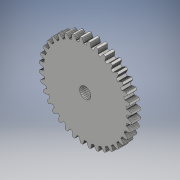
# Autodesk Inventor part: Engranajes GRANDE final 2017
Saved by Autodesk Inventor 2017 (Build 210142000, 142)
## iProperties
Created: 2017-09-25
Part Number: Engranajes GRANDE final 2017
Material: Generic
Document SubType Name: Modeling
Designer: ANDRES
Density: 1 g/cm^3
Appearance: Default
Author: ANDRES
Autodesk Inventor part; units mm, degrees
(part 1 of 2)
ref_plane "YZ Plane" through (0, 0, 0) normal (1, 0, 0) x (0, 1, 0)
ref_plane "XZ Plane" through (0, 0, 0) normal (0, 1, 0) x (-1, 0, 0)
ref_plane "XY Plane" through (0, 0, 0) normal (0, 0, 1) x (1, 0, 0)
sketch "Sketch1" plane through (0, 0, 0) normal (0, 1, 0) x (-1, 0, 0)
  line L0 (23.3143, 11.8442) -> (23.3436, 11.8386)
  line L1 (23.3436, 11.8386) -> (23.3729, 11.8325)
  line L2 (23.3729, 11.8325) -> (23.4022, 11.8259)
  line L3 (23.4022, 11.8259) -> (23.4314, 11.8189)
  line L4 (23.4314, 11.8189) -> (23.4899, 11.8037)
  line L5 (23.4899, 11.8037) -> (23.5482, 11.7869)
  line L6 (23.5482, 11.7869) -> (23.6648, 11.7495)
  line L7 (23.6648, 11.7495) -> (23.781, 11.7072)
  line L8 (23.781, 11.7072) -> (23.8968, 11.6604)
  line L9 (23.8968, 11.6604) -> (24.0123, 11.6095)
  line L10 (24.0123, 11.6095) -> (24.1274, 11.5547)
  line L11 (24.1274, 11.5547) -> (24.2421, 11.4962)
  line L12 (24.2421, 11.4962) -> (24.3563, 11.434)
  line L13 (24.3563, 11.434) -> (24.47, 11.3684)
  line L14 (24.47, 11.3684) -> (24.4188, 10.8271)
  line L15 (24.4188, 10.8271) -> (24.2948, 10.784)
  line L16 (24.2948, 10.784) -> (24.171, 10.7443)
  line L17 (24.171, 10.7443) -> (24.0474, 10.7083)
  line L18 (24.0474, 10.7083) -> (23.9241, 10.676)
  line L19 (23.9241, 10.676) -> (23.8011, 10.6477)
  line L20 (23.8011, 10.6477) -> (23.6785, 10.6234)
  line L21 (23.6785, 10.6234) -> (23.5564, 10.6037)
  line L22 (23.5564, 10.6037) -> (23.435, 10.5887)
  line L23 (23.435, 10.5887) -> (23.3745, 10.5832)
  line L24 (23.3745, 10.5832) -> (23.3142, 10.5792)
  line L25 (23.3142, 10.5792) -> (23.2842, 10.5778)
  line L26 (23.2842, 10.5778) -> (23.2542, 10.5768)
  line L27 (23.2542, 10.5768) -> (23.2243, 10.5763)
  line L28 (23.2243, 10.5763) -> (23.1944, 10.5763)
  line L29 (23.1944, 10.5763) -> (23.0757, 9.9292)
  line L30 (23.0757, 9.9292) -> (23.1036, 9.9186)
  line L31 (23.1036, 9.9186) -> (23.1314, 9.9075)
  line L32 (23.1314, 9.9075) -> (23.159, 9.896)
  line L33 (23.159, 9.896) -> (23.1866, 9.884)
  line L34 (23.1866, 9.884) -> (23.2415, 9.8588)
  line L35 (23.2415, 9.8588) -> (23.2961, 9.8322)
  line L36 (23.2961, 9.8322) -> (23.4044, 9.7751)
  line L37 (23.4044, 9.7751) -> (23.5115, 9.7133)
  line L38 (23.5115, 9.7133) -> (23.6174, 9.6472)
  line L39 (23.6174, 9.6472) -> (23.7223, 9.577)
  line L40 (23.7223, 9.577) -> (23.8262, 9.503)
  line L41 (23.8262, 9.503) -> (23.9289, 9.4254)
  line L42 (23.9289, 9.4254) -> (24.0306, 9.3443)
  line L43 (24.0306, 9.3443) -> (24.1312, 9.26)
  line L44 (24.1312, 9.26) -> (23.9868, 8.7358)
  line L45 (23.9868, 8.7358) -> (23.8572, 8.7148)
  line L46 (23.8572, 8.7148) -> (23.7284, 8.6973)
  line L47 (23.7284, 8.6973) -> (23.6004, 8.6833)
  line L48 (23.6004, 8.6833) -> (23.4733, 8.6729)
  line L49 (23.4733, 8.6729) -> (23.3473, 8.6663)
  line L50 (23.3473, 8.6663) -> (23.2224, 8.6638)
  line L51 (23.2224, 8.6638) -> (23.0987, 8.6655)
  line L52 (23.0987, 8.6655) -> (22.9765, 8.6718)
  line L53 (22.9765, 8.6718) -> (22.916, 8.6769)
  line L54 (22.916, 8.6769) -> (22.856, 8.6834)
  line L55 (22.856, 8.6834) -> (22.8261, 8.6873)
  line L56 (22.8261, 8.6873) -> (22.7964, 8.6915)
  line L57 (22.7964, 8.6915) -> (22.7669, 8.6962)
  line L58 (22.7669, 8.6962) -> (22.7375, 8.7014)
  line L59 (22.7375, 8.7014) -> (22.5082, 8.0848)
  line L60 (22.5082, 8.0848) -> (22.5338, 8.0695)
  line L61 (22.5338, 8.0695) -> (22.5592, 8.0537)
  line L62 (22.5592, 8.0537) -> (22.5845, 8.0375)
  line L63 (22.5845, 8.0375) -> (22.6096, 8.0209)
  line L64 (22.6096, 8.0209) -> (22.6593, 7.9866)
  line L65 (22.6593, 7.9866) -> (22.7084, 7.951)
  line L66 (22.7084, 7.951) -> (22.8051, 7.8759)
  line L67 (22.8051, 7.8759) -> (22.8998, 7.7964)
  line L68 (22.8998, 7.7964) -> (22.9927, 7.7129)
  line L69 (22.9927, 7.7129) -> (23.0838, 7.6255)
  line L70 (23.0838, 7.6255) -> (23.1732, 7.5347)
  line L71 (23.1732, 7.5347) -> (23.2609, 7.4404)
  line L72 (23.2609, 7.4404) -> (23.347, 7.343)
  line L73 (23.347, 7.343) -> (23.4314, 7.2424)
  line L74 (23.4314, 7.2424) -> (23.1982, 6.7513)
  line L75 (23.1982, 6.7513) -> (23.0669, 6.7531)
  line L76 (23.0669, 6.7531) -> (22.937, 6.7582)
  line L77 (22.937, 6.7582) -> (22.8085, 6.7666)
  line L78 (22.8085, 6.7666) -> (22.6816, 6.7786)
  line L79 (22.6816, 6.7786) -> (22.5564, 6.7939)
  line L80 (22.5564, 6.7939) -> (22.4329, 6.8131)
  line L81 (22.4329, 6.8131) -> (22.3114, 6.8362)
  line L82 (22.3114, 6.8362) -> (22.1922, 6.8637)
  line L83 (22.1922, 6.8637) -> (22.1335, 6.8792)
  line L84 (22.1335, 6.8792) -> (22.0755, 6.8961)
  line L85 (22.0755, 6.8961) -> (22.0467, 6.905)
  line L86 (22.0467, 6.905) -> (22.0182, 6.9144)
  line L87 (22.0182, 6.9144) -> (21.9899, 6.9241)
  line L88 (21.9899, 6.9241) -> (21.9619, 6.9343)
  line L89 (21.9619, 6.9343) -> (21.6289, 6.3669)
  line L90 (21.6289, 6.3669) -> (21.6515, 6.3474)
  line L91 (21.6515, 6.3474) -> (21.6738, 6.3275)
  line L92 (21.6738, 6.3275) -> (21.6958, 6.3071)
  line L93 (21.6958, 6.3071) -> (21.7177, 6.2864)
  line L94 (21.7177, 6.2864) -> (21.7607, 6.244)
  line L95 (21.7607, 6.244) -> (21.8029, 6.2003)
  line L96 (21.8029, 6.2003) -> (21.885, 6.1096)
  line L97 (21.885, 6.1096) -> (21.9645, 6.0149)
  line L98 (21.9645, 6.0149) -> (22.0415, 5.9165)
  line L99 (22.0415, 5.9165) -> (22.116, 5.8147)
  line L100 (22.116, 5.8147) -> (22.1883, 5.7097)
  line L101 (22.1883, 5.7097) -> (22.2583, 5.6016)
  line L102 (22.2583, 5.6016) -> (22.3262, 5.4907)
  line L103 (22.3262, 5.4907) -> (22.3918, 5.377)
  line L104 (22.3918, 5.377) -> (22.0769, 4.9338)
  line L105 (22.0769, 4.9338) -> (21.9479, 4.9585)
  line L106 (21.9479, 4.9585) -> (21.8209, 4.986)
  line L107 (21.8209, 4.986) -> (21.6958, 5.0166)
  line L108 (21.6958, 5.0166) -> (21.5729, 5.0503)
  line L109 (21.5729, 5.0503) -> (21.4522, 5.0873)
  line L110 (21.4522, 5.0873) -> (21.3339, 5.1277)
  line L111 (21.3339, 5.1277) -> (21.2183, 5.1716)
  line L112 (21.2183, 5.1716) -> (21.1056, 5.2194)
  line L113 (21.1056, 5.2194) -> (21.0505, 5.2449)
  line L114 (21.0505, 5.2449) -> (20.9963, 5.2715)
  line L115 (20.9963, 5.2715) -> (20.9696, 5.2853)
  line L116 (20.9696, 5.2853) -> (20.9431, 5.2995)
  line L117 (20.9431, 5.2995) -> (20.917, 5.314)
  line L118 (20.917, 5.314) -> (20.8911, 5.3289)
  line L119 (20.8911, 5.3289) -> (20.4647, 4.828)
  line L120 (20.4647, 4.828) -> (20.4835, 4.8049)
  line L121 (20.4835, 4.8049) -> (20.502, 4.7814)
  line L122 (20.502, 4.7814) -> (20.5202, 4.7575)
  line L123 (20.5202, 4.7575) -> (20.5381, 4.7333)
  line L124 (20.5381, 4.7333) -> (20.5731, 4.6841)
  line L125 (20.5731, 4.6841) -> (20.6071, 4.6338)
  line L126 (20.6071, 4.6338) -> (20.6722, 4.5302)
  line L127 (20.6722, 4.5302) -> (20.7341, 4.423)
  line L128 (20.7341, 4.423) -> (20.7928, 4.3127)
  line L129 (20.7928, 4.3127) -> (20.8485, 4.1995)
  line L130 (20.8485, 4.1995) -> (20.9015, 4.0835)
  line L131 (20.9015, 4.0835) -> (20.9517, 3.9649)
  line L132 (20.9517, 3.9649) -> (20.9992, 3.8439)
  line L133 (20.9992, 3.8439) -> (21.0441, 3.7205)
  line L134 (21.0441, 3.7205) -> (20.657, 3.3388)
  line L135 (20.657, 3.3388) -> (20.5343, 3.3854)
  line L136 (20.5343, 3.3854) -> (20.4139, 3.4347)
  line L137 (20.4139, 3.4347) -> (20.2961, 3.4865)
  line L138 (20.2961, 3.4865) -> (20.1809, 3.5411)
  line L139 (20.1809, 3.5411) -> (20.0684, 3.5985)
  line L140 (20.0684, 3.5985) -> (19.959, 3.6587)
  line L141 (19.959, 3.6587) -> (19.8528, 3.722)
  line L142 (19.8528, 3.722) -> (19.7501, 3.7887)
  line L143 (19.7501, 3.7887) -> (19.7002, 3.8233)
  line L144 (19.7002, 3.8233) -> (19.6515, 3.859)
  line L145 (19.6515, 3.859) -> (19.6276, 3.8772)
  line L146 (19.6276, 3.8772) -> (19.604, 3.8957)
  line L147 (19.604, 3.8957) -> (19.5807, 3.9146)
  line L148 (19.5807, 3.9146) -> (19.5578, 3.9338)
  line L149 (19.5578, 3.9338) -> (19.051, 3.5144)
  line L150 (19.051, 3.5144) -> (19.0655, 3.4884)
  line L151 (19.0655, 3.4884) -> (19.0796, 3.462)
  line L152 (19.0796, 3.462) -> (19.0933, 3.4354)
  line L153 (19.0933, 3.4354) -> (19.1068, 3.4084)
  line L154 (19.1068, 3.4084) -> (19.1326, 3.3539)
  line L155 (19.1326, 3.3539) -> (19.1574, 3.2984)
  line L156 (19.1574, 3.2984) -> (19.2036, 3.1851)
  line L157 (19.2036, 3.1851) -> (19.2458, 3.0689)
  line L158 (19.2458, 3.0689) -> (19.2845, 2.9501)
  line L159 (19.2845, 2.9501) -> (19.3198, 2.8289)
  line L160 (19.3198, 2.8289) -> (19.3517, 2.7055)
  line L161 (19.3517, 2.7055) -> (19.3806, 2.58)
  line L162 (19.3806, 2.58) -> (19.4064, 2.4526)
  line L163 (19.4064, 2.4526) -> (19.4292, 2.3233)
  line L164 (19.4292, 2.3233) -> (18.9817, 2.0146)
  line L165 (18.9817, 2.0146) -> (18.8689, 2.0818)
  line L166 (18.8689, 2.0818) -> (18.759, 2.1512)
  line L167 (18.759, 2.1512) -> (18.6519, 2.2227)
  line L168 (18.6519, 2.2227) -> (18.5479, 2.2964)
  line L169 (18.5479, 2.2964) -> (18.4471, 2.3724)
  line L170 (18.4471, 2.3724) -> (18.3498, 2.4507)
  line L171 (18.3498, 2.4507) -> (18.2562, 2.5315)
  line L172 (18.2562, 2.5315) -> (18.1667, 2.615)
  line L173 (18.1667, 2.615) -> (18.1236, 2.6578)
  line L174 (18.1236, 2.6578) -> (18.0818, 2.7013)
  line L175 (18.0818, 2.7013) -> (18.0614, 2.7234)
  line L176 (18.0614, 2.7234) -> (18.0413, 2.7458)
  line L177 (18.0413, 2.7458) -> (18.0217, 2.7684)
  line L178 (18.0217, 2.7684) -> (18.0025, 2.7912)
  line L179 (18.0025, 2.7912) -> (17.4305, 2.4663)
  line L180 (17.4305, 2.4663) -> (17.4403, 2.4381)
  line L181 (17.4403, 2.4381) -> (17.4497, 2.4097)
  line L182 (17.4497, 2.4097) -> (17.4586, 2.381)
  line L183 (17.4586, 2.381) -> (17.4672, 2.3522)
  line L184 (17.4672, 2.3522) -> (17.4832, 2.294)
  line L185 (17.4832, 2.294) -> (17.4979, 2.235)
  line L186 (17.4979, 2.235) -> (17.5237, 2.1154)
  line L187 (17.5237, 2.1154) -> (17.5452, 1.9936)
  line L188 (17.5452, 1.9936) -> (17.5626, 1.8699)
  line L189 (17.5626, 1.8699) -> (17.5763, 1.7445)
  line L190 (17.5763, 1.7445) -> (17.5864, 1.6174)
  line L191 (17.5864, 1.6174) -> (17.593, 1.4888)
  line L192 (17.593, 1.4888) -> (17.5963, 1.3588)
  line L193 (17.5963, 1.3588) -> (17.5963, 1.2275)
  line L194 (17.5963, 1.2275) -> (17.102, 1.0013)
  line L195 (17.102, 1.0013) -> (17.0026, 1.0871)
  line L196 (17.0026, 1.0871) -> (16.9063, 1.1745)
  line L197 (16.9063, 1.1745) -> (16.8133, 1.2636)
  line L198 (16.8133, 1.2636) -> (16.7237, 1.3542)
  line L199 (16.7237, 1.3542) -> (16.6378, 1.4465)
  line L200 (16.6378, 1.4465) -> (16.5555, 1.5406)
  line L201 (16.5555, 1.5406) -> (16.4774, 1.6364)
  line L202 (16.4774, 1.6364) -> (16.4037, 1.7341)
  line L203 (16.4037, 1.7341) -> (16.3687, 1.7838)
  line L204 (16.3687, 1.7838) -> (16.3351, 1.8339)
  line L205 (16.3351, 1.8339) -> (16.3188, 1.8593)
  line L206 (16.3188, 1.8593) -> (16.303, 1.8847)
  line L207 (16.303, 1.8847) -> (16.2876, 1.9104)
  line L208 (16.2876, 1.9104) -> (16.2726, 1.9362)
  line L209 (16.2726, 1.9362) -> (15.6529, 1.7156)
  line L210 (15.6529, 1.7156) -> (15.6577, 1.6861)
  line L211 (15.6577, 1.6861) -> (15.6619, 1.6565)
  line L212 (15.6619, 1.6565) -> (15.6658, 1.6267)
  line L213 (15.6658, 1.6267) -> (15.6692, 1.5968)
  line L214 (15.6692, 1.5968) -> (15.6749, 1.5367)
  line L215 (15.6749, 1.5367) -> (15.6791, 1.4761)
  line L216 (15.6791, 1.4761) -> (15.6838, 1.3538)
  line L217 (15.6838, 1.3538) -> (15.6837, 1.2302)
  line L218 (15.6837, 1.2302) -> (15.6794, 1.1053)
  line L219 (15.6794, 1.1053) -> (15.6711, 0.9794)
  line L220 (15.6711, 0.9794) -> (15.659, 0.8525)
  line L221 (15.659, 0.8525) -> (15.6432, 0.7247)
  line L222 (15.6432, 0.7247) -> (15.6238, 0.5961)
  line L223 (15.6238, 0.5961) -> (15.601, 0.4668)
  line L224 (15.601, 0.4668) -> (15.0749, 0.3298)
  line L225 (15.0749, 0.3298) -> (14.992, 0.4315)
  line L226 (14.992, 0.4315) -> (14.9124, 0.5343)
  line L227 (14.9124, 0.5343) -> (14.8362, 0.6382)
  line L228 (14.8362, 0.6382) -> (14.7637, 0.743)
  line L229 (14.7637, 0.743) -> (14.695, 0.8489)
  line L230 (14.695, 0.8489) -> (14.6303, 0.9558)
  line L231 (14.6303, 0.9558) -> (14.57, 1.0637)
  line L232 (14.57, 1.0637) -> (14.5144, 1.1727)
  line L233 (14.5144, 1.1727) -> (14.4886, 1.2277)
  line L234 (14.4886, 1.2277) -> (14.4642, 1.2829)
  line L235 (14.4642, 1.2829) -> (14.4526, 1.3107)
  line L236 (14.4526, 1.3107) -> (14.4414, 1.3385)
  line L237 (14.4414, 1.3385) -> (14.4307, 1.3665)
  line L238 (14.4307, 1.3665) -> (14.4204, 1.3945)
  line L239 (14.4204, 1.3945) -> (13.7718, 1.2848)
  line L240 (13.7718, 1.2848) -> (13.7714, 1.255)
  line L241 (13.7714, 1.255) -> (13.7705, 1.2251)
  line L242 (13.7705, 1.2251) -> (13.7691, 1.1951)
  line L243 (13.7691, 1.1951) -> (13.7672, 1.1651)
  line L244 (13.7672, 1.1651) -> (13.7624, 1.1049)
  line L245 (13.7624, 1.1049) -> (13.756, 1.0445)
  line L246 (13.756, 1.0445) -> (13.7394, 0.9232)
  line L247 (13.7394, 0.9232) -> (13.7179, 0.8014)
  line L248 (13.7179, 0.8014) -> (13.692, 0.6792)
  line L249 (13.692, 0.6792) -> (13.6619, 0.5567)
  line L250 (13.6619, 0.5567) -> (13.6279, 0.4338)
  line L251 (13.6279, 0.4338) -> (13.5902, 0.3107)
  line L252 (13.5902, 0.3107) -> (13.5488, 0.1874)
  line L253 (13.5488, 0.1874) -> (13.5039, 0.0641)
  line L254 (13.5039, 0.0641) -> (12.962, 0.0205)
  line L255 (12.962, 0.0205) -> (12.8978, 0.1351)
  line L256 (12.8978, 0.1351) -> (12.8373, 0.2501)
  line L257 (12.8373, 0.2501) -> (12.7803, 0.3656)
  line L258 (12.7803, 0.3656) -> (12.7271, 0.4814)
  line L259 (12.7271, 0.4814) -> (12.678, 0.5976)
  line L260 (12.678, 0.5976) -> (12.6328, 0.7141)
  line L261 (12.6328, 0.7141) -> (12.5922, 0.8309)
  line L262 (12.5922, 0.8309) -> (12.5563, 0.9479)
  line L263 (12.5563, 0.9479) -> (12.5404, 1.0065)
  line L264 (12.5404, 1.0065) -> (12.526, 1.0652)
  line L265 (12.526, 1.0652) -> (12.5194, 1.0945)
  line L266 (12.5194, 1.0945) -> (12.5132, 1.1239)
  line L267 (12.5132, 1.1239) -> (12.5075, 1.1533)
  line L268 (12.5075, 1.1533) -> (12.5023, 1.1827)
  line L269 (12.5023, 1.1827) -> (11.8445, 1.1873)
  line L270 (11.8445, 1.1873) -> (11.8389, 1.158)
  line L271 (11.8389, 1.158) -> (11.8328, 1.1287)
  line L272 (11.8328, 1.1287) -> (11.8262, 1.0994)
  line L273 (11.8262, 1.0994) -> (11.8192, 1.0701)
  line L274 (11.8192, 1.0701) -> (11.804, 1.0117)
  line L275 (11.804, 1.0117) -> (11.7872, 0.9533)
  line L276 (11.7872, 0.9533) -> (11.7498, 0.8368)
  line L277 (11.7498, 0.8368) -> (11.7075, 0.7206)
  line L278 (11.7075, 0.7206) -> (11.6607, 0.6047)
  line L279 (11.6607, 0.6047) -> (11.6098, 0.4893)
  line L280 (11.6098, 0.4893) -> (11.555, 0.3742)
  line L281 (11.555, 0.3742) -> (11.4965, 0.2595)
  line L282 (11.4965, 0.2595) -> (11.4343, 0.1453)
  line L283 (11.4343, 0.1453) -> (11.3687, 0.0316)
  line L284 (11.3687, 0.0316) -> (10.8274, 0.0829)
  line L285 (10.8274, 0.0829) -> (10.7843, 0.2068)
  line L286 (10.7843, 0.2068) -> (10.7446, 0.3307)
  line L287 (10.7446, 0.3307) -> (10.7086, 0.4543)
  line L288 (10.7086, 0.4543) -> (10.6763, 0.5776)
  line L289 (10.6763, 0.5776) -> (10.648, 0.7006)
  line L290 (10.648, 0.7006) -> (10.6237, 0.8231)
  line L291 (10.6237, 0.8231) -> (10.604, 0.9452)
  line L292 (10.604, 0.9452) -> (10.589, 1.0667)
  line L293 (10.589, 1.0667) -> (10.5835, 1.1272)
  line L294 (10.5835, 1.1272) -> (10.5795, 1.1874)
  line L295 (10.5795, 1.1874) -> (10.5781, 1.2175)
  line L296 (10.5781, 1.2175) -> (10.5771, 1.2475)
  line L297 (10.5771, 1.2475) -> (10.5766, 1.2774)
  line L298 (10.5766, 1.2774) -> (10.5766, 1.3072)
  line L299 (10.5766, 1.3072) -> (9.9295, 1.426)
  line L300 (9.9295, 1.426) -> (9.9189, 1.3981)
  line L301 (9.9189, 1.3981) -> (9.9078, 1.3703)
  line L302 (9.9078, 1.3703) -> (9.8963, 1.3426)
  line L303 (9.8963, 1.3426) -> (9.8843, 1.315)
  line L304 (9.8843, 1.315) -> (9.8591, 1.2601)
  line L305 (9.8591, 1.2601) -> (9.8325, 1.2055)
  line L306 (9.8325, 1.2055) -> (9.7754, 1.0973)
  line L307 (9.7754, 1.0973) -> (9.7135, 0.9902)
  line L308 (9.7135, 0.9902) -> (9.6474, 0.8842)
  line L309 (9.6474, 0.8842) -> (9.5772, 0.7793)
  line L310 (9.5772, 0.7793) -> (9.5032, 0.6755)
  line L311 (9.5032, 0.6755) -> (9.4257, 0.5727)
  line L312 (9.4257, 0.5727) -> (9.3446, 0.4711)
  line L313 (9.3446, 0.4711) -> (9.2603, 0.3705)
  line L314 (9.2603, 0.3705) -> (8.7361, 0.5149)
  line L315 (8.7361, 0.5149) -> (8.7151, 0.6445)
  line L316 (8.7151, 0.6445) -> (8.6976, 0.7733)
  line L317 (8.6976, 0.7733) -> (8.6836, 0.9013)
  line L318 (8.6836, 0.9013) -> (8.6732, 1.0283)
  line L319 (8.6732, 1.0283) -> (8.6666, 1.1544)
  line L320 (8.6666, 1.1544) -> (8.6641, 1.2793)
  line L321 (8.6641, 1.2793) -> (8.6658, 1.4029)
  line L322 (8.6658, 1.4029) -> (8.6721, 1.5251)
  line L323 (8.6721, 1.5251) -> (8.6772, 1.5856)
  line L324 (8.6772, 1.5856) -> (8.6837, 1.6457)
  line L325 (8.6837, 1.6457) -> (8.6876, 1.6755)
  line L326 (8.6876, 1.6755) -> (8.6918, 1.7052)
  line L327 (8.6918, 1.7052) -> (8.6965, 1.7348)
  line L328 (8.6965, 1.7348) -> (8.7017, 1.7642)
  line L329 (8.7017, 1.7642) -> (8.0851, 1.9935)
  line L330 (8.0851, 1.9935) -> (8.0698, 1.9679)
  line L331 (8.0698, 1.9679) -> (8.054, 1.9424)
  line L332 (8.054, 1.9424) -> (8.0378, 1.9172)
  line L333 (8.0378, 1.9172) -> (8.0212, 1.8921)
  line L334 (8.0212, 1.8921) -> (7.9869, 1.8424)
  line L335 (7.9869, 1.8424) -> (7.9513, 1.7932)
  line L336 (7.9513, 1.7932) -> (7.8762, 1.6966)
  line L337 (7.8762, 1.6966) -> (7.7967, 1.6018)
  line L338 (7.7967, 1.6018) -> (7.7132, 1.509)
  line L339 (7.7132, 1.509) -> (7.6258, 1.4178)
  line L340 (7.6258, 1.4178) -> (7.535, 1.3284)
  line L341 (7.535, 1.3284) -> (7.4407, 1.2407)
  line L342 (7.4407, 1.2407) -> (7.3433, 1.1547)
  line L343 (7.3433, 1.1547) -> (7.2427, 1.0703)
  line L344 (7.2427, 1.0703) -> (6.7516, 1.3034)
  line L345 (6.7516, 1.3034) -> (6.7534, 1.4347)
  line L346 (6.7534, 1.4347) -> (6.7585, 1.5646)
  line L347 (6.7585, 1.5646) -> (6.7669, 1.6931)
  line L348 (6.7669, 1.6931) -> (6.7788, 1.82)
  line L349 (6.7788, 1.82) -> (6.7942, 1.9453)
  line L350 (6.7942, 1.9453) -> (6.8134, 2.0688)
  line L351 (6.8134, 2.0688) -> (6.8365, 2.1902)
  line L352 (6.8365, 2.1902) -> (6.864, 2.3095)
  line L353 (6.864, 2.3095) -> (6.8795, 2.3682)
  line L354 (6.8795, 2.3682) -> (6.8964, 2.4262)
  line L355 (6.8964, 2.4262) -> (6.9053, 2.4549)
  line L356 (6.9053, 2.4549) -> (6.9147, 2.4834)
  line L357 (6.9147, 2.4834) -> (6.9244, 2.5117)
  line L358 (6.9244, 2.5117) -> (6.9346, 2.5398)
  line L359 (6.9346, 2.5398) -> (6.3672, 2.8727)
  line L360 (6.3672, 2.8727) -> (6.3477, 2.8501)
  line L361 (6.3477, 2.8501) -> (6.3278, 2.8278)
  line L362 (6.3278, 2.8278) -> (6.3074, 2.8057)
  line L363 (6.3074, 2.8057) -> (6.2867, 2.7839)
  line L364 (6.2867, 2.7839) -> (6.2443, 2.7409)
  line L365 (6.2443, 2.7409) -> (6.2006, 2.6987)
  line L366 (6.2006, 2.6987) -> (6.1099, 2.6165)
  line L367 (6.1099, 2.6165) -> (6.0152, 2.537)
  line L368 (6.0152, 2.537) -> (5.9168, 2.4601)
  line L369 (5.9168, 2.4601) -> (5.815, 2.3855)
  line L370 (5.815, 2.3855) -> (5.71, 2.3132)
  line L371 (5.71, 2.3132) -> (5.6019, 2.2432)
  line L372 (5.6019, 2.2432) -> (5.491, 2.1754)
  line L373 (5.491, 2.1754) -> (5.3773, 2.1097)
  line L374 (5.3773, 2.1097) -> (4.9341, 2.4247)
  line L375 (4.9341, 2.4247) -> (4.9588, 2.5536)
  line L376 (4.9588, 2.5536) -> (4.9863, 2.6807)
  line L377 (4.9863, 2.6807) -> (5.0169, 2.8058)
  line L378 (5.0169, 2.8058) -> (5.0506, 2.9287)
  line L379 (5.0506, 2.9287) -> (5.0876, 3.0494)
  line L380 (5.0876, 3.0494) -> (5.1279, 3.1676)
  line L381 (5.1279, 3.1676) -> (5.1718, 3.2832)
  line L382 (5.1718, 3.2832) -> (5.2196, 3.3959)
  line L383 (5.2196, 3.3959) -> (5.2451, 3.451)
  line L384 (5.2451, 3.451) -> (5.2717, 3.5052)
  line L385 (5.2717, 3.5052) -> (5.2855, 3.5319)
  line L386 (5.2855, 3.5319) -> (5.2997, 3.5584)
  line L387 (5.2997, 3.5584) -> (5.3142, 3.5846)
  line L388 (5.3142, 3.5846) -> (5.3291, 3.6104)
  line L389 (5.3291, 3.6104) -> (4.8282, 4.0369)
  line L390 (4.8282, 4.0369) -> (4.8051, 4.018)
  line L391 (4.8051, 4.018) -> (4.7816, 3.9995)
  line L392 (4.7816, 3.9995) -> (4.7577, 3.9813)
  line L393 (4.7577, 3.9813) -> (4.7335, 3.9634)
  line L394 (4.7335, 3.9634) -> (4.6843, 3.9285)
  line L395 (4.6843, 3.9285) -> (4.634, 3.8945)
  line L396 (4.634, 3.8945) -> (4.5304, 3.8293)
  line L397 (4.5304, 3.8293) -> (4.4233, 3.7675)
  line L398 (4.4233, 3.7675) -> (4.313, 3.7088)
  line L399 (4.313, 3.7088) -> (4.1998, 3.653)
  line L400 (4.1998, 3.653) -> (4.0838, 3.6001)
  line L401 (4.0838, 3.6001) -> (3.9652, 3.5499)
  line L402 (3.9652, 3.5499) -> (3.8442, 3.5024)
  line L403 (3.8442, 3.5024) -> (3.7208, 3.4575)
  line L404 (3.7208, 3.4575) -> (3.3391, 3.8446)
  line L405 (3.3391, 3.8446) -> (3.3857, 3.9673)
  line L406 (3.3857, 3.9673) -> (3.435, 4.0876)
  line L407 (3.435, 4.0876) -> (3.4868, 4.2055)
  line L408 (3.4868, 4.2055) -> (3.5414, 4.3207)
  line L409 (3.5414, 4.3207) -> (3.5987, 4.4331)
  line L410 (3.5987, 4.4331) -> (3.6589, 4.5426)
  line L411 (3.6589, 4.5426) -> (3.7222, 4.6488)
  line L412 (3.7222, 4.6488) -> (3.7889, 4.7515)
  line L413 (3.7889, 4.7515) -> (3.8235, 4.8013)
  line L414 (3.8235, 4.8013) -> (3.8592, 4.8501)
  line L415 (3.8592, 4.8501) -> (3.8774, 4.874)
  line L416 (3.8774, 4.874) -> (3.8959, 4.8976)
  line L417 (3.8959, 4.8976) -> (3.9148, 4.9209)
  line L418 (3.9148, 4.9209) -> (3.934, 4.9437)
  line L419 (3.934, 4.9437) -> (3.5146, 5.4506)
  line L420 (3.5146, 5.4506) -> (3.4886, 5.436)
  line L421 (3.4886, 5.436) -> (3.4622, 5.4219)
  line L422 (3.4622, 5.4219) -> (3.4356, 5.4081)
  line L423 (3.4356, 5.4081) -> (3.4086, 5.3947)
  line L424 (3.4086, 5.3947) -> (3.3541, 5.3688)
  line L425 (3.3541, 5.3688) -> (3.2986, 5.3441)
  line L426 (3.2986, 5.3441) -> (3.1853, 5.2979)
  line L427 (3.1853, 5.2979) -> (3.0691, 5.2556)
  line L428 (3.0691, 5.2556) -> (2.9503, 5.2169)
  line L429 (2.9503, 5.2169) -> (2.8291, 5.1817)
  line L430 (2.8291, 5.1817) -> (2.7057, 5.1497)
  line L431 (2.7057, 5.1497) -> (2.5802, 5.1209)
  line L432 (2.5802, 5.1209) -> (2.4528, 5.0951)
  line L433 (2.4528, 5.0951) -> (2.3235, 5.0723)
  line L434 (2.3235, 5.0723) -> (2.0148, 5.5198)
  line L435 (2.0148, 5.5198) -> (2.082, 5.6325)
  line L436 (2.082, 5.6325) -> (2.1514, 5.7425)
  line L437 (2.1514, 5.7425) -> (2.2229, 5.8495)
  line L438 (2.2229, 5.8495) -> (2.2966, 5.9535)
  line L439 (2.2966, 5.9535) -> (2.3726, 6.0543)
  line L440 (2.3726, 6.0543) -> (2.4509, 6.1516)
  line L441 (2.4509, 6.1516) -> (2.5317, 6.2453)
  line L442 (2.5317, 6.2453) -> (2.6152, 6.3348)
  line L443 (2.6152, 6.3348) -> (2.658, 6.3779)
  line L444 (2.658, 6.3779) -> (2.7015, 6.4197)
  line L445 (2.7015, 6.4197) -> (2.7236, 6.4401)
  line L446 (2.7236, 6.4401) -> (2.746, 6.4601)
  line L447 (2.746, 6.4601) -> (2.7686, 6.4797)
  line L448 (2.7686, 6.4797) -> (2.7914, 6.4989)
  line L449 (2.7914, 6.4989) -> (2.4665, 7.0709)
  line L450 (2.4665, 7.0709) -> (2.4383, 7.0611)
  line L451 (2.4383, 7.0611) -> (2.4099, 7.0518)
  line L452 (2.4099, 7.0518) -> (2.3812, 7.0428)
  line L453 (2.3812, 7.0428) -> (2.3524, 7.0343)
  line L454 (2.3524, 7.0343) -> (2.2942, 7.0183)
  line L455 (2.2942, 7.0183) -> (2.2352, 7.0035)
  line L456 (2.2352, 7.0035) -> (2.1156, 6.9777)
  line L457 (2.1156, 6.9777) -> (1.9938, 6.9563)
  line L458 (1.9938, 6.9563) -> (1.8701, 6.9388)
  line L459 (1.8701, 6.9388) -> (1.7447, 6.9252)
  line L460 (1.7447, 6.9252) -> (1.6176, 6.9151)
  line L461 (1.6176, 6.9151) -> (1.489, 6.9085)
  line L462 (1.489, 6.9085) -> (1.359, 6.9052)
  line L463 (1.359, 6.9052) -> (1.2277, 6.9052)
  line L464 (1.2277, 6.9052) -> (1.0014, 7.3996)
  line L465 (1.0014, 7.3996) -> (1.0873, 7.499)
  line L466 (1.0873, 7.499) -> (1.1747, 7.5951)
  line L467 (1.1747, 7.5951) -> (1.2638, 7.6881)
  line L468 (1.2638, 7.6881) -> (1.3544, 7.7777)
  line L469 (1.3544, 7.7777) -> (1.4467, 7.8638)
  line L470 (1.4467, 7.8638) -> (1.5408, 7.946)
  line L471 (1.5408, 7.946) -> (1.6366, 8.0242)
  line L472 (1.6366, 8.0242) -> (1.7343, 8.0979)
  line L473 (1.7343, 8.0979) -> (1.784, 8.1329)
  line L474 (1.784, 8.1329) -> (1.8341, 8.1665)
  line L475 (1.8341, 8.1665) -> (1.8595, 8.1827)
  line L476 (1.8595, 8.1827) -> (1.8849, 8.1986)
  line L477 (1.8849, 8.1986) -> (1.9106, 8.214)
  line L478 (1.9106, 8.214) -> (1.9364, 8.2289)
  line L479 (1.9364, 8.2289) -> (1.7158, 8.8486)
  line L480 (1.7158, 8.8486) -> (1.6863, 8.8439)
  line L481 (1.6863, 8.8439) -> (1.6567, 8.8396)
  line L482 (1.6567, 8.8396) -> (1.6269, 8.8358)
  line L483 (1.6269, 8.8358) -> (1.597, 8.8324)
  line L484 (1.597, 8.8324) -> (1.5369, 8.8267)
  line L485 (1.5369, 8.8267) -> (1.4763, 8.8224)
  line L486 (1.4763, 8.8224) -> (1.354, 8.8178)
  line L487 (1.354, 8.8178) -> (1.2304, 8.8178)
  line L488 (1.2304, 8.8178) -> (1.1055, 8.8221)
  line L489 (1.1055, 8.8221) -> (0.9796, 8.8304)
  line L490 (0.9796, 8.8304) -> (0.8527, 8.8426)
  line L491 (0.8527, 8.8426) -> (0.7249, 8.8584)
  line L492 (0.7249, 8.8584) -> (0.5963, 8.8777)
  line L493 (0.5963, 8.8777) -> (0.467, 8.9005)
  line L494 (0.467, 8.9005) -> (0.33, 9.4266)
  line L495 (0.33, 9.4266) -> (0.4317, 9.5096)
  line L496 (0.4317, 9.5096) -> (0.5345, 9.5892)
  line L497 (0.5345, 9.5892) -> (0.6384, 9.6653)
  line L498 (0.6384, 9.6653) -> (0.7432, 9.7378)
  line L499 (0.7432, 9.7378) -> (0.8491, 9.8065)
  line L500 (0.8491, 9.8065) -> (0.956, 9.8712)
  line L501 (0.956, 9.8712) -> (1.0639, 9.9316)
  line L502 (1.0639, 9.9316) -> (1.1729, 9.9872)
  line L503 (1.1729, 9.9872) -> (1.2279, 10.013)
  line L504 (1.2279, 10.013) -> (1.2831, 10.0374)
  line L505 (1.2831, 10.0374) -> (1.3109, 10.049)
  line L506 (1.3109, 10.049) -> (1.3387, 10.0602)
  line L507 (1.3387, 10.0602) -> (1.3667, 10.0709)
  line L508 (1.3667, 10.0709) -> (1.3947, 10.0811)
  line L509 (1.3947, 10.0811) -> (1.285, 10.7297)
  line L510 (1.285, 10.7297) -> (1.2552, 10.7302)
  line L511 (1.2552, 10.7302) -> (1.2253, 10.7311)
  line L512 (1.2253, 10.7311) -> (1.1953, 10.7325)
  line L513 (1.1953, 10.7325) -> (1.1653, 10.7343)
  line L514 (1.1653, 10.7343) -> (1.1051, 10.7392)
  line L515 (1.1051, 10.7392) -> (1.0447, 10.7455)
  line L516 (1.0447, 10.7455) -> (0.9234, 10.7622)
  line L517 (0.9234, 10.7622) -> (0.8016, 10.7837)
  line L518 (0.8016, 10.7837) -> (0.6794, 10.8096)
  line L519 (0.6794, 10.8096) -> (0.5569, 10.8396)
  line L520 (0.5569, 10.8396) -> (0.434, 10.8736)
  line L521 (0.434, 10.8736) -> (0.3109, 10.9114)
  line L522 (0.3109, 10.9114) -> (0.1876, 10.9528)
  line L523 (0.1876, 10.9528) -> (0.0643, 10.9977)
  line L524 (0.0643, 10.9977) -> (0.0207, 11.5396)
  line L525 (0.0207, 11.5396) -> (0.1353, 11.6036)
  line L526 (0.1353, 11.6036) -> (0.2503, 11.6642)
  line L527 (0.2503, 11.6642) -> (0.3658, 11.7211)
  line L528 (0.3658, 11.7211) -> (0.4816, 11.7743)
  line L529 (0.4816, 11.7743) -> (0.5978, 11.8236)
  line L530 (0.5978, 11.8236) -> (0.7143, 11.8687)
  line L531 (0.7143, 11.8687) -> (0.8311, 11.9094)
  line L532 (0.8311, 11.9094) -> (0.9481, 11.9452)
  line L533 (0.9481, 11.9452) -> (1.0067, 11.9611)
  line L534 (1.0067, 11.9611) -> (1.0654, 11.9755)
  line L535 (1.0654, 11.9755) -> (1.0947, 11.9821)
  line L536 (1.0947, 11.9821) -> (1.1241, 11.9883)
  line L537 (1.1241, 11.9883) -> (1.1535, 11.994)
  line L538 (1.1535, 11.994) -> (1.1829, 11.9992)
  line L539 (1.1829, 11.9992) -> (1.1875, 12.657)
  line L540 (1.1875, 12.657) -> (1.1582, 12.6626)
  line L541 (1.1582, 12.6626) -> (1.1289, 12.6688)
  line L542 (1.1289, 12.6688) -> (1.0996, 12.6753)
  line L543 (1.0996, 12.6753) -> (1.0703, 12.6824)
  line L544 (1.0703, 12.6824) -> (1.0119, 12.6976)
  line L545 (1.0119, 12.6976) -> (0.9535, 12.7143)
  line L546 (0.9535, 12.7143) -> (0.837, 12.7518)
  line L547 (0.837, 12.7518) -> (0.7208, 12.7941)
  line L548 (0.7208, 12.7941) -> (0.6049, 12.8408)
  line L549 (0.6049, 12.8408) -> (0.4895, 12.8917)
  line L550 (0.4895, 12.8917) -> (0.3744, 12.9465)
  line L551 (0.3744, 12.9465) -> (0.2597, 13.0051)
  line L552 (0.2597, 13.0051) -> (0.1455, 13.0672)
  line L553 (0.1455, 13.0672) -> (0.0318, 13.1329)
  line L554 (0.0318, 13.1329) -> (0.083, 13.6741)
  line L555 (0.083, 13.6741) -> (0.2069, 13.7173)
  line L556 (0.2069, 13.7173) -> (0.3308, 13.7569)
  line L557 (0.3308, 13.7569) -> (0.4544, 13.793)
  line L558 (0.4544, 13.793) -> (0.5777, 13.8252)
  line L559 (0.5777, 13.8252) -> (0.7007, 13.8536)
  line L560 (0.7007, 13.8536) -> (0.8232, 13.8778)
  line L561 (0.8232, 13.8778) -> (0.9453, 13.8976)
  line L562 (0.9453, 13.8976) -> (1.0668, 13.9126)
  line L563 (1.0668, 13.9126) -> (1.1273, 13.918)
  line L564 (1.1273, 13.918) -> (1.1875, 13.9221)
  line L565 (1.1875, 13.9221) -> (1.2176, 13.9235)
  line L566 (1.2176, 13.9235) -> (1.2476, 13.9245)
  line L567 (1.2476, 13.9245) -> (1.2775, 13.925)
  line L568 (1.2775, 13.925) -> (1.3073, 13.925)
  line L569 (1.3073, 13.925) -> (1.4261, 14.572)
  line L570 (1.4261, 14.572) -> (1.3982, 14.5826)
  line L571 (1.3982, 14.5826) -> (1.3704, 14.5937)
  line L572 (1.3704, 14.5937) -> (1.3427, 14.6053)
  line L573 (1.3427, 14.6053) -> (1.3151, 14.6173)
  line L574 (1.3151, 14.6173) -> (1.2602, 14.6424)
  line L575 (1.2602, 14.6424) -> (1.2056, 14.669)
  line L576 (1.2056, 14.669) -> (1.0974, 14.7262)
  line L577 (1.0974, 14.7262) -> (0.9903, 14.788)
  line L578 (0.9903, 14.788) -> (0.8843, 14.8542)
  line L579 (0.8843, 14.8542) -> (0.7794, 14.9243)
  line L580 (0.7794, 14.9243) -> (0.6756, 14.9983)
  line L581 (0.6756, 14.9983) -> (0.5728, 15.0759)
  line L582 (0.5728, 15.0759) -> (0.4712, 15.1569)
  line L583 (0.4712, 15.1569) -> (0.3706, 15.2413)
  line L584 (0.3706, 15.2413) -> (0.515, 15.7654)
  line L585 (0.515, 15.7654) -> (0.6446, 15.7864)
  line L586 (0.6446, 15.7864) -> (0.7734, 15.804)
  line L587 (0.7734, 15.804) -> (0.9014, 15.818)
  line L588 (0.9014, 15.818) -> (1.0284, 15.8284)
  line L589 (1.0284, 15.8284) -> (1.1545, 15.8349)
  line L590 (1.1545, 15.8349) -> (1.2794, 15.8375)
  line L591 (1.2794, 15.8375) -> (1.403, 15.8358)
  line L592 (1.403, 15.8358) -> (1.5252, 15.8294)
  line L593 (1.5252, 15.8294) -> (1.5857, 15.8243)
  line L594 (1.5857, 15.8243) -> (1.6458, 15.8178)
  line L595 (1.6458, 15.8178) -> (1.6756, 15.814)
  line L596 (1.6756, 15.814) -> (1.7053, 15.8097)
  line L597 (1.7053, 15.8097) -> (1.7349, 15.805)
  line L598 (1.7349, 15.805) -> (1.7643, 15.7999)
  line L599 (1.7643, 15.7999) -> (1.9936, 16.4165)
  line L600 (1.9936, 16.4165) -> (1.968, 16.4317)
  line L601 (1.968, 16.4317) -> (1.9425, 16.4475)
  line L602 (1.9425, 16.4475) -> (1.9173, 16.4637)
  line L603 (1.9173, 16.4637) -> (1.8922, 16.4803)
  line L604 (1.8922, 16.4803) -> (1.8425, 16.5146)
  line L605 (1.8425, 16.5146) -> (1.7933, 16.5503)
  line L606 (1.7933, 16.5503) -> (1.6967, 16.6253)
  line L607 (1.6967, 16.6253) -> (1.6019, 16.7048)
  line L608 (1.6019, 16.7048) -> (1.5091, 16.7884)
  line L609 (1.5091, 16.7884) -> (1.4179, 16.8757)
  line L610 (1.4179, 16.8757) -> (1.3285, 16.9666)
  line L611 (1.3285, 16.9666) -> (1.2408, 17.0608)
  line L612 (1.2408, 17.0608) -> (1.1548, 17.1583)
  line L613 (1.1548, 17.1583) -> (1.0704, 17.2589)
  line L614 (1.0704, 17.2589) -> (1.3035, 17.75)
  line L615 (1.3035, 17.75) -> (1.4348, 17.7481)
  line L616 (1.4348, 17.7481) -> (1.5647, 17.743)
  line L617 (1.5647, 17.743) -> (1.6932, 17.7346)
  line L618 (1.6932, 17.7346) -> (1.8201, 17.7228)
  line L619 (1.8201, 17.7228) -> (1.9454, 17.7073)
  line L620 (1.9454, 17.7073) -> (2.0689, 17.6882)
  line L621 (2.0689, 17.6882) -> (2.1903, 17.665)
  line L622 (2.1903, 17.665) -> (2.3096, 17.6375)
  line L623 (2.3096, 17.6375) -> (2.3683, 17.622)
  line L624 (2.3683, 17.622) -> (2.4263, 17.6052)
  line L625 (2.4263, 17.6052) -> (2.455, 17.5962)
  line L626 (2.455, 17.5962) -> (2.4835, 17.5869)
  line L627 (2.4835, 17.5869) -> (2.5118, 17.5771)
  line L628 (2.5118, 17.5771) -> (2.5399, 17.5669)
  line L629 (2.5399, 17.5669) -> (2.8728, 18.1343)
  line L630 (2.8728, 18.1343) -> (2.8502, 18.1538)
  line L631 (2.8502, 18.1538) -> (2.8279, 18.1738)
  line L632 (2.8279, 18.1738) -> (2.8058, 18.1941)
  line L633 (2.8058, 18.1941) -> (2.784, 18.2148)
  line L634 (2.784, 18.2148) -> (2.741, 18.2572)
  line L635 (2.741, 18.2572) -> (2.6988, 18.3009)
  line L636 (2.6988, 18.3009) -> (2.6166, 18.3916)
  line L637 (2.6166, 18.3916) -> (2.5371, 18.4863)
  line L638 (2.5371, 18.4863) -> (2.4602, 18.5848)
  line L639 (2.4602, 18.5848) -> (2.3856, 18.6866)
  line L640 (2.3856, 18.6866) -> (2.3133, 18.7916)
  line L641 (2.3133, 18.7916) -> (2.2433, 18.8996)
  line L642 (2.2433, 18.8996) -> (2.1755, 19.0106)
  line L643 (2.1755, 19.0106) -> (2.1098, 19.1243)
  line L644 (2.1098, 19.1243) -> (2.4248, 19.5674)
  line L645 (2.4248, 19.5674) -> (2.5537, 19.5428)
  line L646 (2.5537, 19.5428) -> (2.6808, 19.5152)
  line L647 (2.6808, 19.5152) -> (2.8059, 19.4846)
  line L648 (2.8059, 19.4846) -> (2.9288, 19.4509)
  line L649 (2.9288, 19.4509) -> (3.0495, 19.414)
  line L650 (3.0495, 19.414) -> (3.1677, 19.3737)
  line L651 (3.1677, 19.3737) -> (3.2833, 19.3298)
  line L652 (3.2833, 19.3298) -> (3.396, 19.282)
  line L653 (3.396, 19.282) -> (3.4511, 19.2565)
  line L654 (3.4511, 19.2565) -> (3.5053, 19.2298)
  line L655 (3.5053, 19.2298) -> (3.532, 19.216)
  line L656 (3.532, 19.216) -> (3.5585, 19.2019)
  line L657 (3.5585, 19.2019) -> (3.5847, 19.1874)
  line L658 (3.5847, 19.1874) -> (3.6105, 19.1725)
  line L659 (3.6105, 19.1725) -> (4.0369, 19.6734)
  line L660 (4.0369, 19.6734) -> (4.018, 19.6966)
  line L661 (4.018, 19.6966) -> (3.9995, 19.7201)
  line L662 (3.9995, 19.7201) -> (3.9813, 19.7439)
  line L663 (3.9813, 19.7439) -> (3.9634, 19.7681)
  line L664 (3.9634, 19.7681) -> (3.9285, 19.8174)
  line L665 (3.9285, 19.8174) -> (3.8945, 19.8677)
  line L666 (3.8945, 19.8677) -> (3.8294, 19.9713)
  line L667 (3.8294, 19.9713) -> (3.7676, 20.0784)
  line L668 (3.7676, 20.0784) -> (3.7089, 20.1887)
  line L669 (3.7089, 20.1887) -> (3.6531, 20.3019)
  line L670 (3.6531, 20.3019) -> (3.6002, 20.4179)
  line L671 (3.6002, 20.4179) -> (3.55, 20.5364)
  line L672 (3.55, 20.5364) -> (3.5025, 20.6574)
  line L673 (3.5025, 20.6574) -> (3.4576, 20.7808)
  line L674 (3.4576, 20.7808) -> (3.8447, 21.1625)
  line L675 (3.8447, 21.1625) -> (3.9674, 21.1159)
  line L676 (3.9674, 21.1159) -> (4.0877, 21.0667)
  line L677 (4.0877, 21.0667) -> (4.2056, 21.0148)
  line L678 (4.2056, 21.0148) -> (4.3208, 20.9603)
  line L679 (4.3208, 20.9603) -> (4.4332, 20.903)
  line L680 (4.4332, 20.903) -> (4.5427, 20.8427)
  line L681 (4.5427, 20.8427) -> (4.6489, 20.7794)
  line L682 (4.6489, 20.7794) -> (4.7516, 20.7128)
  line L683 (4.7516, 20.7128) -> (4.8014, 20.6781)
  line L684 (4.8014, 20.6781) -> (4.8502, 20.6425)
  line L685 (4.8502, 20.6425) -> (4.8741, 20.6242)
  line L686 (4.8741, 20.6242) -> (4.8977, 20.6057)
  line L687 (4.8977, 20.6057) -> (4.921, 20.5869)
  line L688 (4.921, 20.5869) -> (4.9438, 20.5677)
  line L689 (4.9438, 20.5677) -> (5.4506, 20.987)
  line L690 (5.4506, 20.987) -> (5.436, 21.0131)
  line L691 (5.436, 21.0131) -> (5.4219, 21.0394)
  line L692 (5.4219, 21.0394) -> (5.4081, 21.0661)
  line L693 (5.4081, 21.0661) -> (5.3947, 21.093)
  line L694 (5.3947, 21.093) -> (5.3688, 21.1476)
  line L695 (5.3688, 21.1476) -> (5.3441, 21.2031)
  line L696 (5.3441, 21.2031) -> (5.2979, 21.3164)
  line L697 (5.2979, 21.3164) -> (5.2556, 21.4326)
  line L698 (5.2556, 21.4326) -> (5.2169, 21.5514)
  line L699 (5.2169, 21.5514) -> (5.1817, 21.6726)
  line L700 (5.1817, 21.6726) -> (5.1497, 21.796)
  line L701 (5.1497, 21.796) -> (5.1209, 21.9215)
  line L702 (5.1209, 21.9215) -> (5.0951, 22.0489)
  line L703 (5.0951, 22.0489) -> (5.0723, 22.1782)
  line L704 (5.0723, 22.1782) -> (5.5198, 22.4869)
  line L705 (5.5198, 22.4869) -> (5.6325, 22.4197)
  line L706 (5.6325, 22.4197) -> (5.7425, 22.3503)
  line L707 (5.7425, 22.3503) -> (5.8495, 22.2788)
  line L708 (5.8495, 22.2788) -> (5.9535, 22.205)
  line L709 (5.9535, 22.205) -> (6.0543, 22.1291)
  line L710 (6.0543, 22.1291) -> (6.1516, 22.0507)
  line L711 (6.1516, 22.0507) -> (6.2453, 21.9699)
  line L712 (6.2453, 21.9699) -> (6.3348, 21.8865)
  line L713 (6.3348, 21.8865) -> (6.3779, 21.8437)
  line L714 (6.3779, 21.8437) -> (6.4197, 21.8001)
  line L715 (6.4197, 21.8001) -> (6.4401, 21.778)
  line L716 (6.4401, 21.778) -> (6.4601, 21.7557)
  line L717 (6.4601, 21.7557) -> (6.4797, 21.7331)
  line L718 (6.4797, 21.7331) -> (6.4989, 21.7102)
  line L719 (6.4989, 21.7102) -> (7.0709, 22.0352)
  line L720 (7.0709, 22.0352) -> (7.0611, 22.0633)
  line L721 (7.0611, 22.0633) -> (7.0518, 22.0918)
  line L722 (7.0518, 22.0918) -> (7.0428, 22.1204)
  line L723 (7.0428, 22.1204) -> (7.0343, 22.1493)
  line L724 (7.0343, 22.1493) -> (7.0183, 22.2075)
  line L725 (7.0183, 22.2075) -> (7.0035, 22.2664)
  line L726 (7.0035, 22.2664) -> (6.9777, 22.386)
  line L727 (6.9777, 22.386) -> (6.9563, 22.5078)
  line L728 (6.9563, 22.5078) -> (6.9388, 22.6315)
  line L729 (6.9388, 22.6315) -> (6.9252, 22.757)
  line L730 (6.9252, 22.757) -> (6.9151, 22.8841)
  line L731 (6.9151, 22.8841) -> (6.9085, 23.0126)
  line L732 (6.9085, 23.0126) -> (6.9052, 23.1426)
  line L733 (6.9052, 23.1426) -> (6.9052, 23.2739)
  line L734 (6.9052, 23.2739) -> (7.3995, 23.5002)
  line L735 (7.3995, 23.5002) -> (7.4989, 23.4143)
  line L736 (7.4989, 23.4143) -> (7.5951, 23.3269)
  line L737 (7.5951, 23.3269) -> (7.6881, 23.2379)
  line L738 (7.6881, 23.2379) -> (7.7777, 23.1472)
  line L739 (7.7777, 23.1472) -> (7.8638, 23.0549)
  line L740 (7.8638, 23.0549) -> (7.946, 22.9609)
  line L741 (7.946, 22.9609) -> (8.0242, 22.865)
  line L742 (8.0242, 22.865) -> (8.0979, 22.7673)
  line L743 (8.0979, 22.7673) -> (8.1329, 22.7177)
  line L744 (8.1329, 22.7177) -> (8.1665, 22.6675)
  line L745 (8.1665, 22.6675) -> (8.1827, 22.6422)
  line L746 (8.1827, 22.6422) -> (8.1986, 22.6167)
  line L747 (8.1986, 22.6167) -> (8.214, 22.5911)
  line L748 (8.214, 22.5911) -> (8.2289, 22.5652)
  line L749 (8.2289, 22.5652) -> (8.8486, 22.7859)
  line L750 (8.8486, 22.7859) -> (8.8439, 22.8154)
  line L751 (8.8439, 22.8154) -> (8.8396, 22.845)
  line L752 (8.8396, 22.845) -> (8.8358, 22.8747)
  line L753 (8.8358, 22.8747) -> (8.8324, 22.9046)
  line L754 (8.8324, 22.9046) -> (8.8267, 22.9648)
  line L755 (8.8267, 22.9648) -> (8.8224, 23.0253)
  line L756 (8.8224, 23.0253) -> (8.8178, 23.1476)
  line L757 (8.8178, 23.1476) -> (8.8178, 23.2713)
  line L758 (8.8178, 23.2713) -> (8.8221, 23.3962)
  line L759 (8.8221, 23.3962) -> (8.8304, 23.5221)
  line L760 (8.8304, 23.5221) -> (8.8426, 23.649)
  line L761 (8.8426, 23.649) -> (8.8584, 23.7768)
  line L762 (8.8584, 23.7768) -> (8.8777, 23.9053)
  line L763 (8.8777, 23.9053) -> (8.9005, 24.0346)
  line L764 (8.9005, 24.0346) -> (9.4266, 24.1717)
  line L765 (9.4266, 24.1717) -> (9.5096, 24.0699)
  line L766 (9.5096, 24.0699) -> (9.5892, 23.9671)
  line L767 (9.5892, 23.9671) -> (9.6653, 23.8633)
  line L768 (9.6653, 23.8633) -> (9.7378, 23.7584)
  line L769 (9.7378, 23.7584) -> (9.8065, 23.6526)
  line L770 (9.8065, 23.6526) -> (9.8712, 23.5457)
  line L771 (9.8712, 23.5457) -> (9.9316, 23.4377)
  line L772 (9.9316, 23.4377) -> (9.9872, 23.3287)
  line L773 (9.9872, 23.3287) -> (10.013, 23.2738)
  line L774 (10.013, 23.2738) -> (10.0374, 23.2185)
  line L775 (10.0374, 23.2185) -> (10.049, 23.1908)
  line L776 (10.049, 23.1908) -> (10.0602, 23.1629)
  line L777 (10.0602, 23.1629) -> (10.0709, 23.135)
  line L778 (10.0709, 23.135) -> (10.0811, 23.1069)
  line L779 (10.0811, 23.1069) -> (10.7297, 23.2166)
  line L780 (10.7297, 23.2166) -> (10.7302, 23.2465)
  line L781 (10.7302, 23.2465) -> (10.7311, 23.2764)
  line L782 (10.7311, 23.2764) -> (10.7325, 23.3064)
  line L783 (10.7325, 23.3064) -> (10.7343, 23.3364)
  line L784 (10.7343, 23.3364) -> (10.7392, 23.3966)
  line L785 (10.7392, 23.3966) -> (10.7455, 23.457)
  line L786 (10.7455, 23.457) -> (10.7622, 23.5782)
  line L787 (10.7622, 23.5782) -> (10.7837, 23.7)
  line L788 (10.7837, 23.7) -> (10.8096, 23.8222)
  line L789 (10.8096, 23.8222) -> (10.8396, 23.9448)
  line L790 (10.8396, 23.9448) -> (10.8736, 24.0677)
  line L791 (10.8736, 24.0677) -> (10.9114, 24.1907)
  line L792 (10.9114, 24.1907) -> (10.9528, 24.314)
  line L793 (10.9528, 24.314) -> (10.9977, 24.4374)
  line L794 (10.9977, 24.4374) -> (11.5396, 24.481)
  line L795 (11.5396, 24.481) -> (11.6036, 24.3664)
  line L796 (11.6036, 24.3664) -> (11.6642, 24.2513)
  line L797 (11.6642, 24.2513) -> (11.7211, 24.1358)
  line L798 (11.7211, 24.1358) -> (11.7743, 24.02)
  line L799 (11.7743, 24.02) -> (11.8236, 23.9038)
  line L800 (11.8236, 23.9038) -> (11.8687, 23.7873)
  line L801 (11.8687, 23.7873) -> (11.9094, 23.6705)
  line L802 (11.9094, 23.6705) -> (11.9452, 23.5535)
  line L803 (11.9452, 23.5535) -> (11.9611, 23.4949)
  line L804 (11.9611, 23.4949) -> (11.9755, 23.4363)
  line L805 (11.9755, 23.4363) -> (11.9821, 23.4069)
  line L806 (11.9821, 23.4069) -> (11.9883, 23.3775)
  line L807 (11.9883, 23.3775) -> (11.994, 23.3482)
  line L808 (11.994, 23.3482) -> (11.9992, 23.3188)
  line L809 (11.9992, 23.3188) -> (12.657, 23.3142)
  line L810 (12.657, 23.3142) -> (12.6626, 23.3435)
  line L811 (12.6626, 23.3435) -> (12.6688, 23.3728)
  line L812 (12.6688, 23.3728) -> (12.6753, 23.4021)
  line L813 (12.6753, 23.4021) -> (12.6824, 23.4313)
  line L814 (12.6824, 23.4313) -> (12.6976, 23.4898)
  line L815 (12.6976, 23.4898) -> (12.7143, 23.5481)
  line L816 (12.7143, 23.5481) -> (12.7518, 23.6647)
  line L817 (12.7518, 23.6647) -> (12.7941, 23.7809)
  line L818 (12.7941, 23.7809) -> (12.8408, 23.8967)
  line L819 (12.8408, 23.8967) -> (12.8917, 24.0122)
  line L820 (12.8917, 24.0122) -> (12.9465, 24.1273)
  line L821 (12.9465, 24.1273) -> (13.0051, 24.242)
  line L822 (13.0051, 24.242) -> (13.0672, 24.3562)
  line L823 (13.0672, 24.3562) -> (13.1329, 24.4699)
  line L824 (13.1329, 24.4699) -> (13.6741, 24.4187)
  line L825 (13.6741, 24.4187) -> (13.7173, 24.2947)
  line L826 (13.7173, 24.2947) -> (13.7569, 24.1709)
  line L827 (13.7569, 24.1709) -> (13.793, 24.0473)
  line L828 (13.793, 24.0473) -> (13.8252, 23.924)
  line L829 (13.8252, 23.924) -> (13.8536, 23.801)
  line L830 (13.8536, 23.801) -> (13.8778, 23.6784)
  line L831 (13.8778, 23.6784) -> (13.8976, 23.5563)
  line L832 (13.8976, 23.5563) -> (13.9126, 23.4349)
  line L833 (13.9126, 23.4349) -> (13.918, 23.3744)
  line L834 (13.918, 23.3744) -> (13.9221, 23.3141)
  line L835 (13.9221, 23.3141) -> (13.9235, 23.2841)
  line L836 (13.9235, 23.2841) -> (13.9245, 23.2541)
  line L837 (13.9245, 23.2541) -> (13.925, 23.2242)
  line L838 (13.925, 23.2242) -> (13.925, 23.1943)
  line L839 (13.925, 23.1943) -> (14.572, 23.0756)
  line L840 (14.572, 23.0756) -> (14.5826, 23.1035)
  line L841 (14.5826, 23.1035) -> (14.5937, 23.1313)
  line L842 (14.5937, 23.1313) -> (14.6053, 23.1589)
  line L843 (14.6053, 23.1589) -> (14.6173, 23.1865)
  line L844 (14.6173, 23.1865) -> (14.6424, 23.2414)
  line L845 (14.6424, 23.2414) -> (14.669, 23.296)
  line L846 (14.669, 23.296) -> (14.7262, 23.4043)
  line L847 (14.7262, 23.4043) -> (14.788, 23.5114)
  line L848 (14.788, 23.5114) -> (14.8542, 23.6173)
  line L849 (14.8542, 23.6173) -> (14.9243, 23.7222)
  line L850 (14.9243, 23.7222) -> (14.9983, 23.8261)
  line L851 (14.9983, 23.8261) -> (15.0759, 23.9288)
  line L852 (15.0759, 23.9288) -> (15.1569, 24.0305)
  line L853 (15.1569, 24.0305) -> (15.2413, 24.1311)
  line L854 (15.2413, 24.1311) -> (15.7654, 23.9867)
  line L855 (15.7654, 23.9867) -> (15.7864, 23.8571)
  line L856 (15.7864, 23.8571) -> (15.804, 23.7283)
  line L857 (15.804, 23.7283) -> (15.818, 23.6003)
  line L858 (15.818, 23.6003) -> (15.8284, 23.4732)
  line L859 (15.8284, 23.4732) -> (15.8349, 23.3472)
  line L860 (15.8349, 23.3472) -> (15.8375, 23.2223)
  line L861 (15.8375, 23.2223) -> (15.8358, 23.0986)
  line L862 (15.8358, 23.0986) -> (15.8294, 22.9764)
  line L863 (15.8294, 22.9764) -> (15.8243, 22.9159)
  line L864 (15.8243, 22.9159) -> (15.8178, 22.8559)
  line L865 (15.8178, 22.8559) -> (15.814, 22.826)
  line L866 (15.814, 22.826) -> (15.8097, 22.7963)
  line L867 (15.8097, 22.7963) -> (15.805, 22.7668)
  line L868 (15.805, 22.7668) -> (15.7999, 22.7374)
  line L869 (15.7999, 22.7374) -> (16.4165, 22.5081)
  line L870 (16.4165, 22.5081) -> (16.4317, 22.5337)
  line L871 (16.4317, 22.5337) -> (16.4475, 22.5591)
  line L872 (16.4475, 22.5591) -> (16.4637, 22.5844)
  line L873 (16.4637, 22.5844) -> (16.4803, 22.6095)
  line L874 (16.4803, 22.6095) -> (16.5146, 22.6592)
  line L875 (16.5146, 22.6592) -> (16.5503, 22.7083)
  line L876 (16.5503, 22.7083) -> (16.6253, 22.805)
  line L877 (16.6253, 22.805) -> (16.7048, 22.8997)
  line L878 (16.7048, 22.8997) -> (16.7884, 22.9926)
  line L879 (16.7884, 22.9926) -> (16.8757, 23.0837)
  line L880 (16.8757, 23.0837) -> (16.9666, 23.1731)
  line L881 (16.9666, 23.1731) -> (17.0608, 23.2608)
  line L882 (17.0608, 23.2608) -> (17.1583, 23.3469)
  line L883 (17.1583, 23.3469) -> (17.2589, 23.4313)
  line L884 (17.2589, 23.4313) -> (17.75, 23.1981)
  line L885 (17.75, 23.1981) -> (17.7481, 23.0668)
  line L886 (17.7481, 23.0668) -> (17.743, 22.9369)
  line L887 (17.743, 22.9369) -> (17.7346, 22.8084)
  line L888 (17.7346, 22.8084) -> (17.7228, 22.6815)
  line L889 (17.7228, 22.6815) -> (17.7073, 22.5563)
  line L890 (17.7073, 22.5563) -> (17.6882, 22.4328)
  line L891 (17.6882, 22.4328) -> (17.6651, 22.3113)
  line L892 (17.6651, 22.3113) -> (17.6376, 22.1921)
  line L893 (17.6376, 22.1921) -> (17.6221, 22.1334)
  line L894 (17.6221, 22.1334) -> (17.6053, 22.0754)
  line L895 (17.6053, 22.0754) -> (17.5963, 22.0466)
  line L896 (17.5963, 22.0466) -> (17.587, 22.0181)
  line L897 (17.587, 22.0181) -> (17.5772, 21.9898)
  line L898 (17.5772, 21.9898) -> (17.567, 21.9618)
  line L899 (17.567, 21.9618) -> (18.1344, 21.6289)
  line L900 (18.1344, 21.6289) -> (18.1539, 21.6515)
  line L901 (18.1539, 21.6515) -> (18.1739, 21.6738)
  line L902 (18.1739, 21.6738) -> (18.1942, 21.6958)
  line L903 (18.1942, 21.6958) -> (18.2149, 21.7177)
  line L904 (18.2149, 21.7177) -> (18.2573, 21.7607)
  line L905 (18.2573, 21.7607) -> (18.301, 21.8029)
  line L906 (18.301, 21.8029) -> (18.3917, 21.885)
  line L907 (18.3917, 21.885) -> (18.4864, 21.9645)
  line L908 (18.4864, 21.9645) -> (18.5849, 22.0415)
  line L909 (18.5849, 22.0415) -> (18.6867, 22.116)
  line L910 (18.6867, 22.116) -> (18.7917, 22.1883)
  line L911 (18.7917, 22.1883) -> (18.8997, 22.2583)
  line L912 (18.8997, 22.2583) -> (19.0107, 22.3262)
  line L913 (19.0107, 22.3262) -> (19.1244, 22.3918)
  line L914 (19.1244, 22.3918) -> (19.5674, 22.0768)
  line L915 (19.5674, 22.0768) -> (19.5428, 21.9479)
  line L916 (19.5428, 21.9479) -> (19.5152, 21.8209)
  line L917 (19.5152, 21.8209) -> (19.4846, 21.6958)
  line L918 (19.4846, 21.6958) -> (19.4509, 21.5729)
  line L919 (19.4509, 21.5729) -> (19.414, 21.4522)
  line L920 (19.414, 21.4522) -> (19.3737, 21.3339)
  line L921 (19.3737, 21.3339) -> (19.3298, 21.2183)
  line L922 (19.3298, 21.2183) -> (19.282, 21.1056)
  line L923 (19.282, 21.1056) -> (19.2565, 21.0505)
  line L924 (19.2565, 21.0505) -> (19.2298, 20.9963)
  line L925 (19.2298, 20.9963) -> (19.216, 20.9696)
  line L926 (19.216, 20.9696) -> (19.2019, 20.9431)
  line L927 (19.2019, 20.9431) -> (19.1874, 20.917)
  line L928 (19.1874, 20.917) -> (19.1725, 20.8911)
  line L929 (19.1725, 20.8911) -> (19.6734, 20.4647)
  line L930 (19.6734, 20.4647) -> (19.6966, 20.4835)
  line L931 (19.6966, 20.4835) -> (19.7201, 20.502)
  line L932 (19.7201, 20.502) -> (19.7439, 20.5202)
  line L933 (19.7439, 20.5202) -> (19.7681, 20.5381)
  line L934 (19.7681, 20.5381) -> (19.8174, 20.5731)
  line L935 (19.8174, 20.5731) -> (19.8677, 20.6071)
  line L936 (19.8677, 20.6071) -> (19.9713, 20.6722)
  line L937 (19.9713, 20.6722) -> (20.0784, 20.7341)
  line L938 (20.0784, 20.7341) -> (20.1887, 20.7928)
  line L939 (20.1887, 20.7928) -> (20.3019, 20.8485)
  line L940 (20.3019, 20.8485) -> (20.4179, 20.9015)
  line L941 (20.4179, 20.9015) -> (20.5364, 20.9517)
  line L942 (20.5364, 20.9517) -> (20.6574, 20.9992)
  line L943 (20.6574, 20.9992) -> (20.7808, 21.0441)
  line L944 (20.7808, 21.0441) -> (21.1625, 20.657)
  line L945 (21.1625, 20.657) -> (21.1159, 20.5343)
  line L946 (21.1159, 20.5343) -> (21.0667, 20.4139)
  line L947 (21.0667, 20.4139) -> (21.0148, 20.2961)
  line L948 (21.0148, 20.2961) -> (20.9603, 20.1809)
  line L949 (20.9603, 20.1809) -> (20.903, 20.0684)
  line L950 (20.903, 20.0684) -> (20.8427, 19.959)
  line L951 (20.8427, 19.959) -> (20.7794, 19.8528)
  line L952 (20.7794, 19.8528) -> (20.7128, 19.7501)
  line L953 (20.7128, 19.7501) -> (20.6781, 19.7002)
  line L954 (20.6781, 19.7002) -> (20.6425, 19.6515)
  line L955 (20.6425, 19.6515) -> (20.6242, 19.6276)
  line L956 (20.6242, 19.6276) -> (20.6057, 19.604)
  line L957 (20.6057, 19.604) -> (20.5869, 19.5807)
  line L958 (20.5869, 19.5807) -> (20.5677, 19.5578)
  line L959 (20.5677, 19.5578) -> (20.9869, 19.051)
  line L960 (20.9869, 19.051) -> (21.013, 19.0655)
  line L961 (21.013, 19.0655) -> (21.0393, 19.0797)
  line L962 (21.0393, 19.0797) -> (21.066, 19.0934)
  line L963 (21.066, 19.0934) -> (21.0929, 19.1069)
  line L964 (21.0929, 19.1069) -> (21.1475, 19.1327)
  line L965 (21.1475, 19.1327) -> (21.203, 19.1575)
  line L966 (21.203, 19.1575) -> (21.3164, 19.2037)
  line L967 (21.3164, 19.2037) -> (21.4326, 19.2459)
  line L968 (21.4326, 19.2459) -> (21.5514, 19.2846)
  line L969 (21.5514, 19.2846) -> (21.6726, 19.3199)
  line L970 (21.6726, 19.3199) -> (21.796, 19.3518)
  line L971 (21.796, 19.3518) -> (21.9215, 19.3807)
  line L972 (21.9215, 19.3807) -> (22.0489, 19.4065)
  line L973 (22.0489, 19.4065) -> (22.1782, 19.4293)
  line L974 (22.1782, 19.4293) -> (22.4868, 18.9817)